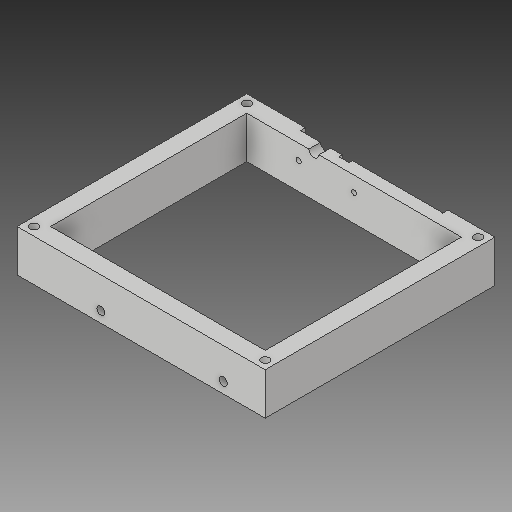
# Autodesk Inventor part: Корпус низ
Saved by Autodesk Inventor 2017 (Build 210142000, 142)
## iProperties
Part Number: Корпус низ
Material: Типовые
Document SubType Name: Modeling
Designer: Daemon
Density: 1 g/cm^3
Appearance: По умолчанию
Author: Daemon
Autodesk Inventor part; units mm, degrees
ref_plane "YZ Plane" through (0, 0, 0) normal (1, 0, 0) x (0, 1, 0)
ref_plane "XZ Plane" through (0, 0, 0) normal (0, 1, 0) x (-1, 0, 0)
sketch "Эскиз1" plane through (0, 0, 0) normal (0, 1, 0) x (-1, 0, 0)
  line L0 (0, 0) -> (148, 0)
  line L1 (148, 0) -> (148, -137)
  line L2 (148, -137) -> (0, -137)
  line L3 (0, -137) -> (0, 0)
  line L4 (10, -10) -> (138, -10)
  line L5 (138, -10) -> (138, -127)
  line L6 (138, -127) -> (10, -127)
  line L7 (10, -127) -> (10, -10)
  line L8 (0, 0) -> (5.5771, 0)
  dimension "d0" = 148
  dimension "d2" = 10
  dimension "d3" = 10
  dimension "d4" = 10
  dimension "d5" = 10
  dimension "d8" = 117
  constraints: 18 end point, 4 parallel, 2 horizontal, 2 perpendicular, 1 point on line
  measures "d0" distance of L1.end L2.end
  measures "d2" distance between parallel lines of L2 L6
  measures "d3" distance between parallel lines of L0 L4
  measures "d4" distance between parallel lines of L1 L5
  measures "d5" distance between parallel lines of L7 L3
  measures "d8" distance between parallel lines of L6 L4
extrude "Выдавливание1" add sketch "Эскиз1" along normal blind 25
sketch "Эскиз2" plane through (0, 25, 0) normal (0, 1, 0) x (1, 0, 0)
  line L0 (0, 0) -> (0, 137) projected
  line L1 (-148, 0) -> (0, 0) projected
  line L2 (0, 5) -> (-148, 5)
  line L3 (-148, 137) -> (-148, 0) projected
  line L4 (-143, 0) -> (-148, 0)
  line L5 (-143, 0) -> (-143, 137)
  line L6 (0, 137) -> (-148, 137) projected
  circle A0 centre (-143, 5) radius 2.5
  dimension "d9" = 5
  dimension "d12" = 5
  dimension "d20" = 5
  constraints: 6 end point, 6 point on line, 1 centre point, 1 collinear, 1 horizontal, 1 vertical
  measures "d9" distance of L0.start L2.start
  measures "d12" distance of L1.start L4.start
  measures "d20" diameter of A0
extrude "Выдавливание2" cut sketch "Эскиз2" against normal through all contours A0 L5 L2 | L2 L5 A0 | A0 L2 L5 | L2 A0 L5
sketch "Эскиз6" plane through (0, 25, 0) normal (0, 1, 0) x (1, 0, 0)
  line L0 (-98, 137) -> (-98, 127)
  line L1 (-138, 127) -> (-10, 127) projected
  line L2 (-148, 137) -> (-148, 0) projected
  line L3 (-98, 127) -> (-101, 127)
  line L4 (-101, 137) -> (-101, 127)
  line L5 (-101, 137) -> (-98, 137)
  line L6 (0, 137) -> (-148, 137) projected
  point P0 (0, 0)
  dimension "d46" = 50
  dimension "d47" = 6
  dimension "d86" = 10
  constraints: 8 end point, 2 point on line, 2 vertical, 1 collinear
  measures "d46" distance between parallel lines of L2 L0
  measures "d47" diameter of L4 L0
  measures "d86" distance of L4.start L3.end
revolve "Вращение3" cut sketch "Эскиз6" angle 360 about axis through (-98, 25, -137) along (0, 0, 1)
sketch "Эскиз8" plane through (0, 25, 0) normal (0, 1, 0) x (1, 0, 0)
  circle A0 centre (-143, 5) radius 2.5 projected
  line L0 (-143, 5) -> (-48, 5)
  circle A1 centre (-5, 5) radius 2.5
  line L1 (0, 0) -> (0, 137) projected
  dimension "d56" = 5
  dimension "d57" = 5
  constraints: 2 end point, 1 centre point, 1 horizontal, 1 point on line
  measures "d56" distance from line of L1 A1.centre
  measures "d57" diameter of A1
extrude "Выдавливание4" cut sketch "Эскиз8" against normal through all contours A1
sketch "Эскиз9" plane through (0, 25, 0) normal (0, 1, 0) x (1, 0, 0)
  circle A0 centre (-5, 5) radius 2.5 projected
  line L0 (-5, 5) -> (-5, 137)
  line L1 (0, 137) -> (-148, 137) projected
  circle A1 centre (-5, 132) radius 2.5
  point P0 (0, 0)
  point P1 (0, 137)
  point P2 (-85.5, 143)
  dimension "d60" = 5
  dimension "d61" = 5
  constraints: 2 end point, 1 centre point, 1 point on line, 1 vertical, 2 other
  measures "d61" diameter of A1
extrude "Выдавливание5" cut sketch "Эскиз9" against normal through all contours A1 L0 | L0 A1
sketch "Эскиз10" plane through (0, 25, 0) normal (0, 1, 0) x (1, 0, 0)
  circle A0 centre (-143, 5) radius 2.5 projected
  line L0 (-143, 5) -> (-143, 137)
  line L1 (-148, 137) -> (0, 137) projected
  circle A1 centre (-5, 132) radius 2.5 projected
  line L2 (-5, 132) -> (-148, 132)
  line L3 (-148, 0) -> (-148, 137) projected
  circle A2 centre (-143, 132) radius 2.5
  point P0 (0, 0)
  dimension "d64" = 5
  constraints: 4 end point, 4 point on line, 1 centre point, 1 horizontal, 1 vertical
  measures "d64" diameter of A2
extrude "Выдавливание6" cut sketch "Эскиз10" against normal through all contours A2 L2 L0 | L0 L2 A2 | L2 A2 L0 | L0 A2 L2
sketch "Эскиз11" plane through (-10, 0, -10) normal (0, 0, -1) x (-1, 0, 0)
  line L0 (0, 25) -> (128, 25) projected
  circle A0 centre (88, 25) radius 18.5
  line L1 (128, 0) -> (0, 0) projected
  circle A1 centre (88, 6.5) radius 2.4
  line L2 (88, 25) -> (88, 6.5)
  line L3 (88, 25) -> (69.5, 25)
  point P0 (-10, 0)
  point P1 (-10, 25)
  point P2 (138, 25)
  dimension "d67" = 37
  dimension "d69" = 4.8
  dimension "d79" = 50
  dimension "d85" = 90
  constraints: 4 end point, 2 centre point, 2 point on circle, 1 point on line
  measures "d67" diameter of A0
  measures "d69" diameter of A1
  measures "d79" distance of point (138, 25) L2.start
  measures "d85" angle of L0 L2
extrude "Выдавливание7" cut sketch "Эскиз11" against normal through all contours A1 L2 A0 | A0 A1 | A1 A0 L2
pattern_linear "Прямоуг.массив3" count 2 spacing -73 along (-1, 0, 0) of "Выдавливание7"
ref_plane "РабПлоскость1" through (0, 0, -68.5) normal (0, 0, 1) x (1, 0, 0)
mirror "Зеркальное отражение1" about plane through (0, 0, -68.5) normal (0, 0, 1) of "Прямоуг.массив3"
sketch "Эскиз14" plane through (0, 0, -137) normal (0, 0, -1) x (-1, 0, 0)
  arc A0 (95, 25) -> (101, 25) centre (98, 25) ccw projected
  line L0 (113, 9) -> (113, 25)
  line L1 (138, 25) -> (101, 25) projected
  line L2 (113, 25) -> (28, 25)
  line L3 (0, 25) -> (95, 25) projected
  line L4 (28, 25) -> (28, 9)
  line L5 (28, 9) -> (113, 9)
  point P0 (0, 0)
  point P1 (148, 25)
  dimension "d89" = 85
  dimension "d90" = 16
  dimension "d91" = 35
  constraints: 8 end point, 2 point on line, 1 horizontal, 1 parallel, 1 vertical
  measures "d89" distance of L0.end L2.end
  measures "d90" distance of L0.start L0.end
  measures "d91" distance from line of point (148, 25) L0
extrude "Выдавливание8" cut sketch "Эскиз14" against normal blind 3 contours A0 L1 L0 L5 L4 L2
sketch "Эскиз15" plane through (0, 0, -134) normal (0, 0, -1) x (-1, 0, 0)
  arc A0 (95, 25) -> (101, 25) centre (98, 25) ccw projected
  line L0 (148, 25) -> (0, 25) projected
  line L1 (113, 9) -> (107, 9)
  line L2 (113, 9) -> (28, 9) projected
  line L3 (107, 9) -> (107, 16)
  circle A1 centre (107, 16) radius 1.5
  point P0 (0, 0)
  dimension "d98" = 6
  dimension "d99" = 7
  dimension "d100" = 3
  constraints: 4 end point, 1 centre point, 1 coincident, 1 point on line, 1 vertical
  measures "d98" distance of L1.start L1.end
  measures "d99" distance of L1.end L3.end
  measures "d100" diameter of A1
extrude "Выдавливание9" cut sketch "Эскиз15" against normal up to next contours A1
sketch "Эскиз16" plane through (0, 0, -134) normal (0, 0, -1) x (-1, 0, 0)
  line L0 (113, 9) -> (28, 9) projected
  circle A0 centre (107, 16) radius 1.5 projected
  line L1 (107, 16) -> (74, 16)
  circle A1 centre (74, 16) radius 1.5
  point P0 (0, 0)
  dimension "d106" = 33
  dimension "d107" = 3
  constraints: 2 end point, 1 centre point, 1 coincident, 1 horizontal
  measures "d106" distance of L1.start L1.end
  measures "d107" diameter of A1
extrude "Выдавливание10" cut sketch "Эскиз16" against normal up to next contours A1
sketch "Эскиз17" plane through (0, 0, -134) normal (0, 0, -1) x (-1, 0, 0)
  circle A0 centre (74, 16) radius 1.5 projected
  circle A1 centre (74, 16) radius 3.7
  point P0 (0, 0)
  dimension "d110" = 7.4
  constraints: 1 centre point, 1 coincident
  measures "d110" diameter of A1
extrude "Выдавливание11" cut sketch "Эскиз17" against normal blind 2
sketch "Эскиз18" plane through (0, 0, -134) normal (0, 0, -1) x (-1, 0, 0)
  circle A0 centre (107, 16) radius 1.5 projected
  circle A1 centre (107, 16) radius 3.7
  point P0 (0, 0)
  dimension "d113" = 7.4
  constraints: 1 centre point, 1 coincident
  measures "d113" diameter of A1
extrude "Выдавливание12" cut sketch "Эскиз18" against normal blind 2
sketch "Эскиз19" plane through (0, 0, -134) normal (0, 0, -1) x (-1, 0, 0)
  arc A0 (82, 20) -> (88, 20) centre (85, 20) ccw
  line L0 (113, 9) -> (28, 9) projected
  line L1 (113, 25) -> (113, 9) projected
  line L2 (10, 25) -> (138, 25) projected
  line L3 (82, 20) -> (82, 25)
  line L4 (88, 20) -> (88, 25)
  point P0 (0, 0)
  dimension "d121" = 6
  dimension "d123" = 25
  dimension "d124" = 11
  constraints: 4 end point, 2 point on circle, 2 point on line, 2 tangent, 1 centre point, 1 perpendicular, 1 vertical
  measures "d121" diameter of A0
  measures "d123" distance between parallel lines of L1 L4
  measures "d124" distance from line of L4.start L0
extrude "Выдавливание13" cut sketch "Эскиз19" against normal blind 2
